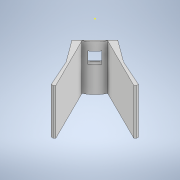
# Autodesk Inventor part: Box_Walls_2
Saved by Autodesk Inventor 2022 (Build 260153000, 153)
## iProperties
Created: 2023-02-27
Part Number: Box_Walls_2
Material: Generic
Document SubType Name: Modeling
Designer: zarek
Density: 1 g/cm^3
Appearance: Default
Author: zarek
Autodesk Inventor part; units mm, degrees
ref_plane "YZ Plane" through (0, 0, 0) normal (1, 0, 0) x (0, 1, 0)
ref_plane "XZ Plane" through (0, 0, 0) normal (0, 1, 0) x (-1, 0, 0)
sketch "Sketch1" plane through (0, 0, 0) normal (0, 1, 0) x (-1, 0, 0)
  line L0 (101.6, -101.6) -> (-101.6, -101.6)
  line L1 (-101.6, -101.6) -> (-101.6, 101.6)
  line L2 (-101.6, 101.6) -> (101.6, 101.6)
  line L3 (101.6, 101.6) -> (101.6, -101.6)
  line L4 (96.6, -96.6) -> (-96.6, -96.6)
  line L5 (-96.6, -96.6) -> (-96.6, 96.6)
  line L6 (-96.6, 96.6) -> (96.6, 96.6)
  line L7 (96.6, 96.6) -> (96.6, -96.6)
  line L8 (101.6, 101.6) -> (-40.4, 101.6)
  circle A0 centre (0, 0) radius 88.9
  circle A1 centre (0, 0) radius 109.3376
  line L9 (-40.4, 101.6) -> (-101.6, 40.4)
  line L10 (-45.4, 101.6) -> (-101.6, 45.4)
  line L11 (96.6, 96.6) -> (96.6, 101.6)
  line L12 (-45.4, 101.6) -> (-35.4, 101.6)
  line L13 (-35.4, 101.6) -> (-35.4, 96.6)
  line L14 (-35.4, 96.6) -> (-45.4, 96.6)
  line L15 (-45.4, 96.6) -> (-45.4, 101.6)
  line L16 (-45.4, 101.6) -> (-43.114, 101.6)
  line L17 (-43.114, 101.6) -> (-43.114, 96.6)
  line L18 (-43.114, 96.6) -> (-45.4, 96.6)
  line L19 (-45.4, 96.6) -> (-45.4, 101.6)
  line L20 (-96.6, 45.4) -> (-101.6, 45.4)
  line L21 (-101.6, 45.4) -> (-101.6, 43.114)
  line L22 (-101.6, 43.114) -> (-96.6, 43.114)
  line L23 (-96.6, 43.114) -> (-96.6, 45.4)
  point P0 (96.6, 51.2168)
  point P1 (101.6, 40.4)
  point P2 (101.6, -40.4)
  point P3 (96.6, -51.2168)
  point P4 (-96.6, 45.4)
  point P5 (-45.4, 96.6)
  dimension "d0" = 203.2
  dimension "d1" = 203.2
  dimension "d2" = 101.6
  dimension "d3" = 101.6
  dimension "d4" = 5
  dimension "d5" = 5
  dimension "d6" = 5
  dimension "d7" = 5
  dimension "d10" = 142
  dimension "d12" = 61.2
  dimension "d14" = 177.8
  dimension "d15" = 5
  dimension "d16" = 5
  dimension "d17" = 10
  dimension "d86" = 2.286
  dimension "d87" = 2.286
  constraints: 48 end point, 11 parallel, 10 point on line, 6 perpendicular, 5 horizontal, 2 centre point, 2 coincident, 2 point on circle
  measures "d0" distance between parallel lines of L2 L0
  measures "d1" distance between parallel lines of L1 L3
  measures "d2" distance from line of L0 point (0, 0)
  measures "d3" distance from line of L1 point (0, 0)
  measures "d4" distance between parallel lines of L4 L0
  measures "d5" distance between parallel lines of L1 L5
  measures "d6" distance between parallel lines of L2 L6
  measures "d7" distance between parallel lines of L3 L7
  measures "d10" distance of L2.end L8.end
  measures "d12" distance from line of L1 L8.end
  measures "d14" diameter of A0
  measures "d15" distance of L10.end L9.end
  measures "d16" distance of L10.start L8.end
  measures "d17" distance of L13.end L14.end
  measures "d86" distance of L17.end L18.end
  measures "d87" distance of L21.end L20.end
extrude "Extrusion1" add sketch "Sketch1" along normal blind 5 contours L0 A1 L4 L7 L3 | L0 A1 L4 | A1 L7 L3 | L0 L1 A1 L5 L4 | A1 L7 L4 | L4 A1 L5 L9 L6 L7 | A1 L7 L11 L2 L3 | L4 L5 A1 | A1 L6 L7 | L1 L9 L22 L5 A1 | L11 L6 A1 L2 | L6 L13 L2 A1 | L1 L22 A1 | A1 L22 L9 | L22 L9 L5 | L6 L17 L9 L2 L13 | L1 L20 A1 L22 | A1 L20 L9 L22 | L20 A1 L10 L5 | L5 L10 L6 L9 | A1 L17 L2 | L9 L17 A1 | L6 L9 L17 | L1 L2 L10 A1 L6 L5 | L10 A1 L20 | L10 A1 L5 | L5 A1 L6 L10 | L15 A1 L17 L9 | L6 L10 A1 L15 | L17 A1 L15 L2 | L5 L6 A1 | L6 A1 L10 | A1 L10 L15 | A0
sketch "Sketch3" plane through (0, 5, 0) normal (0, 1, 0) x (1, 0, 0)
  circle A0 centre (0, 0) radius 88.9
  line L0 (-101.6, 101.6) -> (-101.6, -101.6) projected
  line L1 (-101.6, -101.6) -> (101.6, -101.6) projected
  line L2 (-101.6, 101.6) -> (101.6, 101.6)
  line L3 (101.6, 101.6) -> (101.6, -101.6)
  line L4 (101.6, -101.6) -> (-101.6, -101.6)
  line L5 (-101.6, -101.6) -> (-101.6, 101.6)
  line L6 (-96.6, 96.6) -> (96.6, 96.6)
  line L7 (96.6, 96.6) -> (96.6, -96.6)
  line L8 (96.6, -96.6) -> (-96.6, -96.6)
  line L9 (-96.6, -96.6) -> (-96.6, 96.6)
  line L10 (-101.6, -101.6) -> (40.4, -101.6)
  circle A1 centre (0, 0) radius 109.3376
  line L11 (40.4, -101.6) -> (101.6, -40.4)
  line L12 (101.6, -101.6) -> (101.6, 101.6) projected
  line L13 (45.4038, -101.6) -> (101.6, -45.4038)
  line L14 (96.6, -45.4) -> (101.6, -45.4038)
  line L15 (45.4, -96.6) -> (45.4038, -101.6)
  line L16 (96.6, -45.4) -> (101.6, -45.4)
  line L17 (101.6, -45.4) -> (101.6, -43.114)
  line L18 (101.6, -43.114) -> (96.6, -43.114)
  line L19 (96.6, -43.114) -> (96.6, -45.4)
  line L20 (45.4038, -101.6) -> (43.1178, -101.6)
  line L21 (43.1178, -101.6) -> (43.1178, -96.6)
  line L22 (43.1178, -96.6) -> (45.4038, -96.6)
  line L23 (45.4038, -96.6) -> (45.4038, -101.6)
  point P0 (45.4038, -101.6)
  point P1 (50.4038, -96.6)
  point P2 (96.6, -50.4038)
  dimension "d28" = 177.8
  dimension "d29" = 5
  dimension "d30" = 5
  dimension "d31" = 5
  dimension "d32" = 5
  dimension "d33" = 142
  dimension "d76" = 5.0038
  dimension "d77" = 5.0038
  dimension "d88" = 2.286
  dimension "d89" = 2.286
  constraints: 42 end point, 10 point on line, 9 parallel, 4 horizontal, 4 perpendicular, 2 centre point, 2 coincident, 2 point on circle
  measures "d28" diameter of A0
  measures "d29" distance between parallel lines of L3 L7
  measures "d30" distance between parallel lines of L6 L2
  measures "d31" distance between parallel lines of L0 L9
  measures "d32" distance between parallel lines of L1 L8
  measures "d33" distance of L4.end L10.end
  measures "d76" distance of L13.end L11.end
  measures "d77" distance of L13.start L10.end
  measures "d88" distance of L17.end L16.end
  measures "d89" distance of L21.end L22.end
extrude "Extrusion3" cut sketch "Sketch3" against normal blind 2 contours L2 A1 L6 L9 L0 | A1 L9 L0 | L2 A1 L6 | A1 L9 L8 L1 L0 | L2 L3 A1 L7 L6 | A1 L8 L21 L11 L1 | L3 L11 L18 L7 A1 | A1 L21 L1 | L11 L21 A1 | L3 L18 A1 | A1 L18 L11
sketch "Sketch4" plane through (0, 5, 0) normal (0, 1, 0) x (1, 0, 0)
  line L0 (101.6, 101.6) -> (-101.6, 101.6)
  line L1 (-101.6, 101.6) -> (-101.6, -101.6)
  line L2 (-101.6, -101.6) -> (101.6, -101.6)
  line L3 (101.6, -101.6) -> (101.6, 101.6)
  circle A0 centre (0, 0) radius 2.5
  line L4 (11.3314, 2.139) -> (-2.139, -11.3314)
  line L5 (0, 0) -> (-5.6569, 5.6569)
  line L6 (-5.6569, -14.8492) -> (-26.163, 5.6569)
  line L7 (-5.6569, 26.163) -> (14.8492, 5.6569)
  circle A1 centre (-5.6569, 5.6569) radius 14
  line L8 (-26.163, 5.6569) -> (-5.6569, 26.163)
  line L9 (14.8492, 5.6569) -> (-5.6569, -14.8492)
  line L10 (-40.3051, 5.6569) -> (-5.6569, 40.3051)
  line L11 (-5.6569, 40.3051) -> (28.9914, 5.6569)
  line L12 (28.9914, 5.6569) -> (-5.6569, -28.9914)
  line L13 (-5.6569, -28.9914) -> (-40.3051, 5.6569)
  line L14 (-22.6451, 9.1747) -> (-9.1747, 22.6451)
  line L15 (-9.1747, 22.6451) -> (-12.7668, 26.2372)
  line L16 (-12.7668, 26.2372) -> (-26.2372, 12.7668)
  line L17 (-26.2372, 12.7668) -> (-22.6451, 9.1747)
  point P0 (9.525, 22.5)
  point P1 (-9.525, -6.5)
  dimension "d37" = 203.2
  dimension "d38" = 203.2
  dimension "d39" = 8
  dimension "d40" = 28
  dimension "d41" = 29
  dimension "d42" = 29
  dimension "d43" = 14.5
  dimension "d44" = 10
  dimension "d45" = 10
  dimension "d46" = 10
  dimension "d47" = 10
  dimension "d48" = 5.08
  dimension "d49" = 9.525
  dimension "d50" = 9.525
  dimension "d55" = 101.6
  dimension "d56" = 101.6
  constraints: 36 end point, 8 parallel, 4 perpendicular, 2 centre point, 2 coincident, 2 point on line, 1 horizontal
  measures "d37" distance between parallel lines of L2 L0
  measures "d38" distance between parallel lines of L1 L3
  measures "d39" distance of L5.start L5.end
  measures "d40" diameter of A1
  measures "d41" distance between parallel lines of L9 L8
  measures "d42" distance between parallel lines of L7 L6
  measures "d43" distance from line of A1.centre L8
  measures "d44" distance between parallel lines of L11 L7
  measures "d45" distance between parallel lines of L8 L10
  measures "d46" distance between parallel lines of L13 L6
  measures "d47" distance between parallel lines of L12 L9
  measures "d48" distance between parallel lines of L14 L16
  measures "d49" distance from line of A1.centre L15
  measures "d50" distance from line of L5.end L17
  measures "d55" distance from line of point (0, 0) L1
  measures "d56" distance from line of L0 point (0, 0)
extrude "Extrusion4" cut sketch "Sketch4" against normal blind 1 contours A0 | L4 L9 L6 L8 L7 | L8 L17 L16 L15 | A1 | L10 L11 L12 L13
sketch "Sketch6" plane through (0, 5, 0) normal (0, 1, 0) x (1, 0, 0)
  line L0 (45.4038, -101.6) -> (0, 0)
  line L1 (50.4038, -96.6) -> (45.4038, -101.6) projected
  line L2 (96.6, -43.114) -> (96.6, 96.6) projected
  line L3 (101.6, -101.6) -> (101.6, 101.6) projected
  circle A0 centre (0, 0) radius 34.925
  circle A1 centre (0, 0) radius 33.425
  line L4 (-101.6, 101.6) -> (-101.6, -101.6) projected
  line L5 (-101.6, -101.6) -> (40.4, -101.6)
  line L6 (-101.6, -101.6) -> (101.6, -101.6) projected
  line L7 (101.6, 101.6) -> (101.6, -43.114) projected
  line L8 (101.6, -45.4038) -> (0, 0)
  line L9 (-96.6, -96.6) -> (43.1178, -96.6) projected
  line L10 (96.6, -43.114) -> (96.6, 96.6) projected
  line L11 (43.1178, -101.6) -> (-101.6, -101.6) projected
  line L12 (101.6, -45.4038) -> (96.6, -50.4038) projected
  line L13 (45.4038, -101.6) -> (101.6, -45.4038)
  line L14 (43.1178, -101.6) -> (101.6, -101.6) projected
  line L15 (0, 0) -> (101.6, -50.4076)
  line L16 (50.4076, -101.6) -> (0, 0)
  line L17 (43.1694, -96.6) -> (47.9269, -96.6)
  line L18 (96.6, -43.1694) -> (96.6, -47.9269)
  line L19 (40.4, -101.6) -> (101.6, -40.4)
  point P0 (13.6374, -30.5164)
  point P1 (30.5164, -13.6374)
  point P2 (14.2494, -31.8859)
  point P3 (31.2861, -15.5222)
  point P4 (29.9423, -14.8555)
  point P5 (31.8859, -14.2494)
  point P6 (98.2555, -48.7483)
  point P7 (96.6, -47.9269)
  point P8 (47.9269, -96.6)
  point P9 (15.5222, -31.2861)
  point P10 (96.6, -45.4)
  point P11 (45.4, -96.6)
  point P12 (14.8555, -29.9423)
  point P13 (96.6, -45.4)
  point P14 (45.4, -96.6)
  point P15 (45.4, -96.6)
  point P16 (47.089, -94.911)
  point P17 (94.911, -47.089)
  point P18 (96.6, -45.4)
  point P19 (43.8583, -98.1417)
  point P20 (98.1417, -43.8583)
  point P21 (45.4, -96.6)
  point P22 (96.6, -45.4)
  dimension "d71" = 69.85
  dimension "d72" = 66.85
  dimension "d75" = 142
  dimension "d78" = 5.0038
  dimension "d82" = 5.0038
  constraints: 18 end point, 11 point on line, 2 centre point, 2 coincident, 1 collinear, 1 perpendicular
  measures "d71" diameter of A0
  measures "d72" diameter of A1
  measures "d75" distance of L4.end L5.end
  measures "d78" distance of L0.start L5.end
  measures "d82" distance of L8.start L19.end
extrude "Extrusion6" add sketch "Sketch6" along normal blind 56 contours L0 A0 L16 L19 L17 | L0 A1 L16 A0 | L16 A1 L15 A0 | L15 A0 L8 L18 L19 | A0 L15 A1 L8
fillet "Fillet3" radius 12.7 1 edges at (101.6, 2.5, 101.6)
sketch "Sketch9" plane through (0, 4, 0) normal (0, 1, 0) x (1, 0, 0)
  point P0 (0, 0)
sketch "Sketch10" plane through (0, 5, 0) normal (0, 1, 0) x (1, 0, 0)
  point P0 (0, 0)
ref_plane "Work Plane1" through (24.6957, 5, 24.6957) normal (0.7071068, 0, 0.7071068) x (0.7071068, 0, -0.7071068)
sketch "Sketch15" plane through (0, 5, 0) normal (0, 1, 0) x (1, 0, 0)
  line L0 (13.6374, -30.5164) -> (43.1694, -96.6) projected
  line L1 (28.4034, -63.5582) -> (-0.6569, -23.9914)
  line L2 (28.9914, 5.6569) -> (-5.6569, -28.9914) projected
  line L3 (96.6, -43.1694) -> (30.5164, -13.6374) projected
  line L4 (-5.6569, 40.3051) -> (28.9914, 5.6569) projected
  line L5 (63.5582, -28.4034) -> (23.9914, 0.6569)
  line L6 (2.3374, -28.0682) -> (28.0682, -2.3374)
  arc A0 (13.6374, -30.5164) -> (30.5164, -13.6374) centre (0, 0) ccw projected
  line L7 (28.4034, -63.5582) -> (13.6374, -30.5164)
  line L8 (63.5582, -28.4034) -> (30.5164, -13.6374)
  arc A1 (13.6374, -30.5164) -> (30.5164, -13.6374) centre (0, 0) ccw
  dimension "d138" = 5
  dimension "d139" = 5
  dimension "d140" = 5
  constraints: 10 end point, 4 point on line, 3 point on circle, 2 midpoint, 1 centre point, 1 collinear, 1 concentric, 1 parallel
  measures "d138" horizontal distance of L2.end L1.end
  measures "d139" horizontal distance of L2.start L5.end
  measures "d140" distance between parallel lines of L6 L2
extrude "Extrusion11" add sketch "Sketch15" along normal up to surface (56 mm away) contours L0 L1 L6 L5 L3 A0
sketch "Sketch16" plane through (0, 61, 0) normal (0, 1, 0) x (1, 0, 0)
  line L0 (2.3374, -28.0682) -> (28.0682, -2.3374) projected
  line L1 (9.4085, -20.9971) -> (12.2369, -23.8255)
  line L2 (12.2369, -23.8255) -> (23.8256, -12.2369)
  line L3 (23.8256, -12.2369) -> (20.9971, -9.4085)
  line L4 (12.2369, -23.8255) -> (23.8256, -12.2369)
  line L5 (23.8256, -12.2369) -> (28.5592, -16.9706)
  line L6 (28.5592, -16.9706) -> (16.9706, -28.5592)
  line L7 (16.9706, -28.5592) -> (12.2369, -23.8255)
  line L8 (28.4034, -63.5582) -> (2.3374, -28.0682) projected
  line L9 (28.0682, -2.3374) -> (63.5582, -28.4034) projected
  line L10 (23.8256, -12.2369) -> (31.3296, -4.7328)
  line L11 (12.2369, -23.8255) -> (4.7328, -31.3296)
  line L12 (28.4034, -63.5582) -> (2.3374, -28.0682) projected
  point P0 (0, 0)
  point P1 (29.3133, -3.2519)
  point P2 (12.2369, -23.8255)
  dimension "d144" = 10
  dimension "d145" = 10
  dimension "d146" = 4
  dimension "d152" = 0
  dimension "d153" = 0
  constraints: 18 end point, 6 perpendicular, 6 point on line
  measures "d144" distance of L0.start L1.start
  measures "d145" distance of L0.end L3.end
  measures "d146" distance between parallel lines of L0 L2
  measures "d152" distance between parallel lines of L7 L1
  measures "d153" distance between parallel lines of L5 L3
extrude "Extrusion12" cut sketch "Sketch16" against normal up to surface (56 mm away)
sketch "Sketch11" plane through (24.6957, 5, 24.6957) normal (0.7071068, 0, 0.7071068) x (0.7071068, 0, -0.7071068)
  line L0 (143.6841, -5) -> (0, -5) projected
  line L1 (0, -5) -> (0, 40)
  circle A0 centre (0, 40) radius 5.5
  line L2 (-6, 46) -> (6, 46)
  line L3 (6, 46) -> (6, 34)
  line L4 (6, 34) -> (-6, 34)
  line L5 (-6, 34) -> (-6, 46)
  line L6 (0, 46) -> (0, 56)
  line L7 (8.1944, 56) -> (-8.1944, 56) projected
  dimension "d144" = 10
  dimension "d145" = 10
  dimension "d146" = 4
  dimension "d152" = 0
  dimension "d153" = 0
  dimension "d120" = 45
  dimension "d121" = 11
  dimension "d221" = 6
  dimension "d222" = 6
  dimension "d223" = 6
  dimension "d224" = 6
  dimension "d271" = 10
  constraints: 12 end point, 2 midpoint, 2 parallel, 1 centre point, 1 coincident, 1 horizontal, 1 perpendicular, 1 vertical
  measures "d120" distance of L0.end L1.end
  measures "d121" diameter of A0
  measures "d221" distance from line of L3 L1.end
  measures "d222" distance from line of L5 L1.end
  measures "d223" distance from line of L1.end L2
  measures "d224" distance from line of L4 L1.end
  measures "d271" distance of L6.start L6.end
extrude "Extrusion8" cut sketch "Sketch11" against normal blind 127 contours A0 | L2 L3 L4 L5
sketch "Sketch18" plane through (101.6, 3, 43.114) normal (1, 0, 0) x (0, 0, -1)
  line L0 (-53.486, 2) -> (-58.486, 2) projected
  line L1 (-58.486, 2) -> (145.4353, 2)
  line L2 (145.4353, 2) -> (145.4353, -4.8825)
  line L3 (145.4353, -4.8825) -> (-58.486, -4.8825)
  line L4 (-58.486, -4.8825) -> (-58.486, 2)
  point P0 (43.114, -3)
  constraints: 8 end point, 2 parallel, 1 horizontal, 1 perpendicular
extrude "Extrusion13" cut sketch "Sketch18" against normal through all
sketch "Sketch30" plane through (0, 61, 0) normal (0, 1, 0) x (1, 0, 0)
  line L0 (2.3374, -28.0682) -> (28.0682, -2.3374)
  line L1 (9.4085, -20.9971) -> (12.944, -24.5327)
  line L2 (12.944, -24.5327) -> (24.5327, -12.944)
  line L3 (24.5327, -12.944) -> (20.9971, -9.4085)
  line L4 (12.944, -24.5327) -> (24.5327, -12.944)
  line L5 (24.5327, -12.944) -> (28.5592, -16.9706)
  line L6 (28.5592, -16.9706) -> (16.9706, -28.5592)
  line L7 (16.9706, -28.5592) -> (12.944, -24.5327)
  line L8 (12.944, -24.5327) -> (5.3317, -32.145)
  line L9 (28.4034, -63.5582) -> (2.3374, -28.0682)
  line L10 (24.5327, -12.944) -> (32.145, -5.3317)
  line L11 (28.0682, -2.3374) -> (63.5582, -28.4034)
  line L12 (31.3296, -4.7328) -> (63.5582, -28.4034) projected
  line L13 (36.788, -8.7418) -> (28.5592, -16.9706)
  line L14 (28.5592, -16.9706) -> (8.7418, -36.788)
  line L15 (36.788, -8.7418) -> (32.145, -5.3317)
  line L16 (28.4034, -63.5582) -> (4.7328, -31.3296) projected
  line L17 (8.7418, -36.788) -> (5.3317, -32.145)
  point P0 (0, 0)
  point P1 (0, 0)
  point P2 (16.9706, -28.5592)
  dimension "d231" = 10
  dimension "d232" = 10
  dimension "d233" = 5
  dimension "d234" = 0
  dimension "d235" = 0
  dimension "d240" = 0
  constraints: 32 end point, 10 point on line, 7 perpendicular, 2 collinear
  measures "d231" distance of L0.start L1.start
  measures "d232" distance of L0.end L3.end
  measures "d233" distance between parallel lines of L0 L2
  measures "d234" distance between parallel lines of L7 L1
  measures "d235" distance between parallel lines of L5 L3
  measures "d240" distance between parallel lines of L14 L6
extrude "Extrusion14" cut sketch "Sketch30" against normal blind 24.75 contours L0 L1 L8 L9 | L0 L11 L10 L3 | L7 L14 L9 L8 | L10 L11 L13 L5
sketch "Sketch32" plane through (28.4034, 5, 63.5582) normal (-0.8059719, 0, 0.5919538) x (0.5919538, 0, 0.8059719)
  line L0 (-33.2148, 56) -> (-33.2148, 31.25) projected
  line L1 (-33.2148, 31.25) -> (-38.2681, 31.25)
  line L2 (-41.5932, 31.25) -> (-34.9759, 31.25) projected
  line L3 (-38.9873, 31.25) -> (-33.2148, 43.625)
  point P0 (-68.0396, -5)
  point P1 (-40.6047, 22.75)
  point P2 (-45.5472, 22.75)
  constraints: 4 end point, 1 horizontal, 1 midpoint, 2 other
sketch "Sketch33" plane through (0, 36.25, 0) normal (0, 1, 0) x (1, 0, 0)
  circle A0 centre (2, 3.9204) radius 1.5
  circle A1 centre (33.9053, 3.9204) radius 1.5
  line L0 (35.9053, 0) -> (31.9053, 0)
  line L1 (31.9053, 7.8408) -> (35.9053, 7.8408)
  line L2 (35.9053, 7.8408) -> (35.9053, 0)
  line L3 (31.9053, 2) -> (31.9053, 7.8408)
  line L4 (0, 0) -> (0, 7.8408)
  line L5 (0, 7.8408) -> (4, 7.8408)
  circle A2 centre (31.2131, -8.6598) radius 1.5
  circle A3 centre (8.6529, -31.22) radius 1.5
  line L6 (31.3296, -4.7328) -> (36.788, -8.7418) projected
  line L7 (8.7418, -36.788) -> (4.7328, -31.3296) projected
  line L8 (31.2131, -8.6598) -> (8.6529, -31.22)
  line L9 (36.788, -8.7418) -> (8.7418, -36.788) projected
  line L10 (12.2369, -23.8255) -> (16.9706, -28.5592) projected
  line L11 (28.5592, -16.9706) -> (23.8256, -12.2369) projected
  point P0 (36.9053, 0)
  point P1 (32.145, -5.3317)
  point P2 (5.3317, -32.145)
  point P3 (28.0682, -2.3374)
  point P4 (2.3374, -28.0682)
  dimension "d241" = 3
  dimension "d242" = 3
  dimension "d243" = 7.8408
  dimension "d244" = 3.9204
  dimension "d245" = 4
  dimension "d246" = 2
  dimension "d247" = 2
  dimension "d248" = 3.9204
  dimension "d249" = 31.9053
  dimension "d250" = 3
  dimension "d251" = 3
  dimension "d254" = 31.905
  dimension "d264" = 4
  dimension "d269" = 7.7629
  dimension "d270" = 7.7532
  constraints: 14 end point, 4 centre point, 1 parallel
  measures "d241" diameter of A0
  measures "d242" diameter of A1
  measures "d243" distance between parallel lines of L0 L1
  measures "d244" distance from line of A1.centre L1
  measures "d245" distance between parallel lines of L2 L3
  measures "d246" distance from line of L2 A1.centre
  measures "d247" distance from line of L4 A0.centre
  measures "d248" distance from line of A0.centre L5
  measures "d249" distance of A1.centre A0.centre
  measures "d250" diameter of A2
  measures "d251" diameter of A3
  measures "d254" distance of L8.start L8.end
  measures "d264" distance between parallel lines of L8 L9
  measures "d269" distance from line of L10 L8.end
  measures "d270" distance from line of L11 L8.start
hole "Hole3" at (8.6529, 36.25, 31.22) at (31.2131, 36.25, 8.6598) direction (0, -1, 0) diameter 2.85 depth 12.7 tip angle 118 countersink diameter 3.81 countersink angle 82 thread size "M3.5x0.6" class "6H" standard "ANSI Metric M Profile"
chamfer "Chamfer1" distance 2 distance2 2 1 edges at (24.6957, 39, 24.6957) measured on face at (17.0887, 35, 30.4587)
sketch "Sketch34" plane through (0, 61, 0) normal (0, 1, 0) x (1, 0, 0)
  point P0 (0, 0)
equation "\"d1\" = d0"
equation "\"d2\" = 0.5 * d0"
equation "\"d3\" = 0.5 * d0"
body "Solid1"
